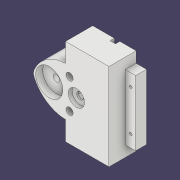
# Autodesk Inventor part: AA006b
Saved by Autodesk Inventor 2017 SP1 (Build 210196100, 196)
## iProperties
Created: 2017-06-04
Part Number: AA006b
Material: ABS Plastic
Document SubType Name: Modeling
Designer: Zach
Density: 1.06 g/cm^3
Appearance: CR White
Author: Zach
Autodesk Inventor part; units mm, degrees
ref_plane "YZ Plane" through (0, 0, 0) normal (1, 0, 0) x (0, 1, 0)
ref_plane "XZ Plane" through (0, 0, 0) normal (0, 1, 0) x (-1, 0, 0)
ref_plane "XY Plane" through (0, 0, 0) normal (0, 0, 1) x (1, 0, 0)
sketch "Sketch1" plane through (0, 0, 0) normal (0, 0, 1) x (1, 0, 0)
  line L0 (0, 0) -> (160, 0)
  line L1 (160, 0) -> (160, 160)
  line L2 (160, 160) -> (0, 160)
  line L3 (0, 160) -> (0, 0)
  circle A0 centre (50, 80) radius 6
  point P0 (160, 80)
  dimension "d0" = 160
  dimension "d1" = 160
  dimension "d2" = 12
  dimension "d7" = 50
  constraints: 8 end point, 2 parallel, 1 centre point, 1 horizontal, 1 horizontal alignment, 1 midpoint, 1 perpendicular
  measures "d0" distance of L2.end L1.end
  measures "d1" distance of L1.end L0.end
  measures "d2" diameter of A0
  measures "d7" distance from line of L3 A0.centre
extrude "Extrusion1" add sketch "Sketch1" along normal blind 50
sketch "Sketch5" plane through (0, 0, 50) normal (0, 0, 1) x (1, 0, 0)
  circle A0 centre (50, 80) radius 6 projected
  line L0 (0, 0) -> (160, 0) projected
  line L1 (160, 0) -> (160, 160) projected
  line L2 (160, 160) -> (0, 160) projected
  line L3 (0, 160) -> (0, 0) projected
  circle A1 centre (80, 80) radius 80 construction
  line L4 (0, 0) -> (160, 0) projected
  arc A2 (80, 160) -> (80, 0) centre (80, 80) ccw
  line L5 (160, 160) -> (0, 160) projected
  line L6 (80, 160) -> (0, 160)
  line L7 (0, 160) -> (0, 0)
  line L8 (80, 0) -> (0, 0)
  point P0 (0, 80)
  constraints: 6 end point, 4 point on circle, 4 tangent, 3 midpoint, 2 centre point, 2 collinear, 1 horizontal alignment, 1 perpendicular
extrude "Extrusion5" cut sketch "Sketch5" against normal through all contours L3 A2 L0 | L3 L2 A2
sketch "Sketch17" plane through (0, 0, 50) normal (0, 0, 1) x (1, 0, 0)
  circle A0 centre (50, 80) radius 6 projected
  circle A1 centre (50, 80) radius 6 projected
  circle A2 centre (50, 80) radius 25
  point P0 (0, 0)
  dimension "d80" = 50
  constraints: 1 centre point, 1 coincident
  measures "d80" diameter of A2
extrude "Extrusion17" cut sketch "Sketch17" against normal blind 10
sketch "Sketch18" plane through (0, 0, 0) normal (0, 0, -1) x (-1, 0, 0)
  circle A0 centre (-50, 80) radius 6 projected
  point P0 (0, 0)
extrude "Extrusion18" add sketch "Sketch18" against normal blind 12.5
sketch "Sketch19" plane through (0, 0, 0) normal (0, 0, -1) x (-1, 0, 0)
  line L0 (-160, 0) -> (-160, 160) projected
  line L1 (-160, 20) -> (-179, 20)
  line L2 (-179, 20) -> (-179, 140)
  line L3 (-179, 140) -> (-160, 140)
  line L4 (-160, 140) -> (-160, 20)
  line L5 (-80, 0) -> (-160, 0) projected
  line L6 (-160, 160) -> (-80, 160) projected
  circle A0 centre (-170, 42.5) radius 2.5
  line L7 (-170, 42.5) -> (-170, 117.5) construction
  circle A1 centre (-170, 117.5) radius 2.5
  point P0 (0, 0)
  point P1 (-160, 80)
  point P2 (-170, 80)
  point P3 (-160, 80)
  dimension "d85" = 19
  dimension "d86" = 20
  dimension "d87" = 20
  dimension "d88" = 5
  dimension "d89" = 10
  dimension "d100" = 75
  dimension "d101" = 5
  constraints: 10 end point, 3 midpoint, 2 centre point, 2 parallel, 1 coincident, 1 horizontal, 1 horizontal alignment, 1 perpendicular, 1 point on line, 1 vertical
  measures "d85" distance of L2.end L3.end
  measures "d86" distance between parallel lines of L1 L5
  measures "d87" distance between parallel lines of L6 L3
  measures "d88" diameter of A0
  measures "d89" distance from line of L0 L7.start
  measures "d100" distance of L7.start L7.end
  measures "d101" diameter of A1
extrude "Extrusion19" add sketch "Sketch19" against normal blind 20
sketch "Sketch20" plane through (0, 0, 0) normal (0, 0, -1) x (-1, 0, 0)
  circle A0 centre (-170, 42.5) radius 2.5 projected
  circle A1 centre (-170, 42.5) radius 6.5
  circle A2 centre (-170, 117.5) radius 2.5 projected
  circle A3 centre (-170, 117.5) radius 6.5
  point P0 (0, 0)
  dimension "d92" = 13
  dimension "d102" = 13
  constraints: 2 centre point, 2 coincident
  measures "d92" diameter of A1
  measures "d102" diameter of A3
extrude "Extrusion20" cut sketch "Sketch20" against normal blind 15 contours A0 | A1 | A3
sketch "Sketch21" plane through (0, 0, 0) normal (0, 0, -1) x (-1, 0, 0)
  circle A0 centre (-170, 42.5) radius 6.5 projected
  arc A1 (-80, 0) -> (-80, 160) centre (-80, 80) ccw projected
  line L0 (-160, 160) -> (-80, 160) projected
  line L1 (-160, 140) -> (-160, 160) projected
  line L2 (-179, 140) -> (-160, 140) projected
  line L3 (-179, 20) -> (-179, 140) projected
  line L4 (-160, 20) -> (-179, 20) projected
  line L5 (-160, 0) -> (-160, 20) projected
  line L6 (-80, 0) -> (-160, 0) projected
  circle A2 centre (-50, 80) radius 6 construction
  arc A3 (-80, 10) -> (-80, 150) centre (-80, 80) ccw construction
  line L7 (-80, 10) -> (-150, 10)
  line L8 (-150, 10) -> (-150, 30)
  line L9 (-150, 30) -> (-169, 30) construction
  line L10 (-169, 30) -> (-169, 130) construction
  line L11 (-169, 130) -> (-150, 130) construction
  line L12 (-150, 130) -> (-150, 150)
  line L13 (-150, 150) -> (-80, 150)
  line L14 (-150, 130) -> (-150, 30) construction
  line L15 (-150, 72.5) -> (-73.8485, 72.5)
  line L16 (-111.9242, 72.5) -> (-111.9242, 87.5) construction
  line L17 (-150, 87.5) -> (-73.8485, 87.5)
  line L18 (-150, 130) -> (-150, 87.5)
  line L19 (-150, 30) -> (-150, 72.5)
  line L20 (-26.1515, 72.5) -> (-10.4029, 72.5)
  line L21 (-26.1515, 87.5) -> (-10.4029, 87.5)
  line L22 (-57.5, 103.8485) -> (-57.5, 146.2854)
  line L23 (-42.5, 103.8485) -> (-42.5, 139.108)
  line L24 (-57.5, 121.4782) -> (-42.5, 121.4782) construction
  line L25 (-42.5, 56.1515) -> (-42.5, 20.892)
  line L26 (-57.5, 56.1515) -> (-57.5, 13.7146)
  circle A4 centre (-50, 80) radius 25 construction
  arc A5 (-57.5, 146.2854) -> (-80, 150) centre (-80, 80) ccw
  arc A6 (-10.4029, 87.5) -> (-42.5, 139.108) centre (-80, 80) ccw
  arc A7 (-42.5, 20.892) -> (-10.4029, 72.5) centre (-80, 80) ccw
  arc A8 (-80, 10) -> (-57.5, 13.7146) centre (-80, 80) ccw
  arc A9 (-57.5, 103.8485) -> (-73.8485, 87.5) centre (-50, 80) ccw
  arc A10 (-26.1515, 87.5) -> (-42.5, 103.8485) centre (-50, 80) ccw
  arc A11 (-42.5, 56.1515) -> (-26.1515, 72.5) centre (-50, 80) ccw
  arc A12 (-73.8485, 72.5) -> (-57.5, 56.1515) centre (-50, 80) ccw
  point P0 (0, 0)
  point P1 (-111.9242, 80)
  point P2 (-50, 121.4782)
  dimension "d95" = 10
  dimension "d96" = 15
  dimension "d99" = 15
  constraints: 40 end point, 27 point on circle, 9 centre point, 9 concentric, 5 midpoint, 5 vertical, 3 horizontal, 3 horizontal alignment, 3 point on line, 3 vertical alignment, 2 collinear, 2 parallel, 1 perpendicular, 7 other
  measures "d95" distance between parallel lines of L0 L13
  measures "d96" distance of L16.end L16.start
  measures "d99" distance of L24.end L24.start
extrude "Extrusion21" cut sketch "Sketch21" against normal blind 40 contours L7 L8 L19 L15 A12 L26 A8 | L12 L13 A5 L22 A9 L17 L18 | L20 A7 L25 A11 | A10 L23 A6 L21
sketch "Sketch23" plane through (0, 0, 50) normal (0, 0, 1) x (1, 0, 0)
  circle A0 centre (87.5, 52.5) radius 2.5
  circle A1 centre (87.5, 107.5) radius 2.5
  line L0 (160, 0) -> (160, 160) construction
  line L1 (87.5, 52.5) -> (87.5, 107.5) construction
  point P0 (0, 0)
  point P1 (87.5, 80)
  point P2 (160, 80)
  dimension "d103" = 5
  dimension "d104" = 5
  dimension "d105" = 55
  dimension "d106" = 72.5
  constraints: 2 centre point, 2 end point, 2 midpoint, 1 horizontal alignment, 1 vertical, 1 vertical alignment
  measures "d103" diameter of A0
  measures "d104" diameter of A1
  measures "d105" distance of L1.start L1.end
  measures "d106" distance from line of L0 L1.start
extrude "Extrusion22" cut sketch "Sketch23" against normal through all
sketch "Sketch24" plane through (0, 0, 40) normal (0, 0, -1) x (-1, 0, 0)
  line L0 (-95, 150) -> (-95, 10)
  line L1 (-80, 150) -> (-80, 10)
  line L2 (-80, 150) -> (-95, 150)
  line L3 (-95, 10) -> (-80, 10)
  line L4 (-95, 80) -> (-80, 80) construction
  circle A0 centre (-87.5, 107.5) radius 2.5 projected
  circle A1 centre (-87.5, 52.5) radius 2.5 projected
  point P0 (0, 0)
  point P1 (-87.5, 80)
  point P2 (-87.5, 10)
  point P3 (-150, 150)
  point P4 (-150, 10)
  dimension "d110" = 15
  constraints: 10 end point, 4 horizontal alignment, 4 midpoint, 2 horizontal, 2 vertical, 1 vertical alignment
  measures "d110" distance of L4.start L4.end
extrude "Extrusion23" add sketch "Sketch24" along normal blind 40
sketch "Sketch26" plane through (0, 0, 50) normal (0, 0, 1) x (1, 0, 0)
  circle A0 centre (87.5, 107.5) radius 2.5 projected
  circle A1 centre (87.5, 52.5) radius 2.5 projected
  circle A2 centre (87.5, 52.5) radius 6.5
  circle A3 centre (87.5, 107.5) radius 6.5
  point P0 (0, 0)
  dimension "d115" = 13
  dimension "d116" = 13
  constraints: 2 centre point, 2 coincident
  measures "d115" diameter of A2
  measures "d116" diameter of A3
extrude "Extrusion24" cut sketch "Sketch26" against normal blind 30 contours A0 | A1 | A2 | A3
sketch "Sketch27" plane through (0, 0, 50) normal (0, 0, 1) x (1, 0, 0)
  arc A0 (80, 160) -> (80, 0) centre (80, 80) ccw construction
  circle A1 centre (80, 80) radius 80 construction
  circle A2 centre (80, 80) radius 60 construction
  line L0 (80, 0) -> (160, 0) projected
  line L1 (160, 160) -> (80, 160) projected
  arc A3 (80, 160) -> (80, 0) centre (80, 80) ccw projected
  arc A4 (80, 160) -> (80, 160) centre (80, 80) ccw
  line L2 (80, 160) -> (80, 140)
  line L3 (160, 0) -> (122.4264, 37.5736)
  line L4 (160, 0) -> (80, 80) construction
  arc A5 (80, 140) -> (122.4264, 37.5736) centre (80, 80) ccw
  circle A6 centre (50, 80) radius 6 projected
  arc A7 (80, 160) -> (80, 0) centre (80, 80) ccw projected
  point P0 (0, 0)
  dimension "d119" = 20
  constraints: 6 end point, 6 point on circle, 3 centre point, 2 coincident, 2 concentric, 2 vertical alignment, 1 point on line, 1 vertical, 6 other
extrude "Extrusion25" cut sketch "Sketch27" against normal blind 25 contours A4 L3 L0 | A3 L2 A5 L3 A4
sketch "Sketch30" plane through (0, 0, 25) normal (0, 0, 1) x (1, 0, 0)
  line L0 (95, 21.9052) -> (95, 10)
  line L1 (122.4264, 37.5736) -> (160, 0) construction
  arc A0 (95, 21.9052) -> (122.4264, 37.5736) centre (80, 80) ccw
  line L2 (150, 10) -> (122.4264, 37.5736)
  arc A1 (80, 140) -> (122.4264, 37.5736) centre (80, 80) ccw projected
  line L3 (95, 10) -> (150, 10) projected
  line L4 (95, 10) -> (150, 10) projected
  point P0 (0, 0)
  constraints: 6 end point, 2 point on circle, 1 centre point, 1 concentric, 1 point on line, 1 vertical
extrude "Extrusion28" add sketch "Sketch30" against normal blind 5
sketch "Sketch31" plane through (0, 0, 25) normal (0, 0, 1) x (1, 0, 0)
  arc A0 (10.4029, 72.5) -> (42.5, 20.892) centre (80, 80) ccw projected
  line L0 (80, 87.5) -> (80, 150) projected
  arc A1 (57.5, 13.7146) -> (80, 10) centre (80, 80) ccw projected
  line L1 (26.1515, 72.5) -> (10.4029, 72.5) projected
  arc A2 (80, 150) -> (80, 10) centre (80, 80) ccw
  arc A3 (80, 140) -> (122.4264, 37.5736) centre (80, 80) ccw projected
  line L2 (80, 10) -> (80, 20)
  line L3 (80, 150) -> (80, 140)
  line L4 (80, 140) -> (80, 20)
  arc A4 (80, 140) -> (80, 20) centre (80, 80) ccw
  constraints: 6 end point, 6 point on circle, 2 centre point, 2 vertical, 1 collinear, 1 concentric
extrude "Extrusion29" add sketch "Sketch31" against normal blind 10 contours L1 A3 L2 A1 A2 A0 | A2 L0 A3 L1
sketch "Sketch32" plane through (0, 0, 40) normal (0, 0, -1) x (-1, 0, 0)
  arc A0 (-122.4264, 37.5736) -> (-80, 140) centre (-80, 80) ccw construction
  line L0 (-122.4264, 37.5736) -> (-160, 0) construction
  line L1 (-160, 0) -> (-160, 160) construction
  arc A1 (-122.2654, 44.8057) -> (-80, 135) centre (-80, 80) ccw construction
  line L2 (-122.2654, 44.8057) -> (-155, 12.0711) construction
  line L3 (-155, 12.0711) -> (-155, 160) construction
  line L4 (-150, 10) -> (-150, 72.5) construction
  arc A2 (-122.4264, 37.5736) -> (-80, 140) centre (-80, 80) ccw
  arc A3 (-122.2654, 44.8057) -> (-80, 135) centre (-80, 80) ccw
  line L5 (-122.2654, 44.8057) -> (-150, 17.0711)
  line L6 (-150, 10) -> (-150, 17.0711)
  line L7 (-150, 10) -> (-122.4264, 37.5736)
  line L8 (-80, 140) -> (-80, 135)
  point P0 (0, 0)
  dimension "d155" = 5
  constraints: 12 end point, 6 point on circle, 3 centre point, 2 collinear, 2 concentric, 2 point on line, 1 parallel, 2 other
  measures "d155" radial gap between concentric circles of A0 A1
extrude "Extrusion30" add sketch "Sketch32" along normal blind 25
sketch "Sketch33" plane through (0, 0, 20) normal (0, 0, -1) x (-1, 0, 0)
  line L0 (-95, 10) -> (-150, 10) projected
  line L1 (-95, 21.9052) -> (-95, 10) projected
  arc A0 (-122.4264, 37.5736) -> (-95, 21.9052) centre (-80, 80) ccw projected
  line L2 (-122.4264, 37.5736) -> (-150, 10) projected
  point P0 (0, 0)
extrude "Extrusion31" add sketch "Sketch33" along normal blind 5
sketch "Sketch34" plane through (0, 0, 50) normal (0, 0, 1) x (1, 0, 0)
  circle A0 centre (100, 80) radius 6.5
  circle A1 centre (50, 80) radius 6 projected
  point P0 (0, 0)
  dimension "d143" = 13
  dimension "d144" = 50
  constraints: 1 centre point, 1 horizontal alignment
  measures "d143" diameter of A0
  measures "d144" distance of A0.centre A1.centre
extrude "Extrusion32" cut sketch "Sketch34" against normal through all contours A0
sketch "Sketch35" plane through (0, 0, 40) normal (0, 0, -1) x (-1, 0, 0)
  line L0 (-88, 94.5) -> (-112, 94.5)
  line L1 (-112, 94.5) -> (-112, 65.5)
  line L2 (-112, 65.5) -> (-88, 65.5)
  line L3 (-88, 65.5) -> (-88, 94.5)
  circle A0 centre (-100, 80) radius 6.5 projected
  line L4 (-95, 55.5) -> (-150, 55.5)
  line L5 (-150, 55.5) -> (-150, 104.5)
  line L6 (-150, 104.5) -> (-95, 104.5)
  line L7 (-95, 104.5) -> (-95, 55.5)
  line L8 (-150, 10) -> (-150, 72.5) projected
  line L9 (-95, 72.5) -> (-95, 10) projected
  point P0 (0, 0)
  point P1 (-88, 80)
  point P2 (-100, 65.5)
  dimension "d147" = 29
  dimension "d148" = 24
  dimension "d153" = 10
  dimension "d154" = 10
  constraints: 16 end point, 4 parallel, 2 midpoint, 2 perpendicular, 2 point on line, 1 horizontal, 1 horizontal alignment, 1 vertical alignment
  measures "d147" distance of L2.end L0.start
  measures "d148" distance of L1.end L2.end
  measures "d153" distance between parallel lines of L4 L2
  measures "d154" distance between parallel lines of L0 L6
extrude "Extrusion33" add sketch "Sketch35" along normal blind 40 contours L0 L1 L2 L7 L4 L5 L6
sketch "Sketch36" plane through (0, 0, 40) normal (0, 0, -1) x (-1, 0, 0)
  line L0 (-112, 94.5) -> (-112, 87.5) construction
  line L1 (-73.8485, 87.5) -> (-80, 87.5) construction
  line L2 (-95, 94.5) -> (-112, 94.5) construction
  line L3 (-112, 72.5) -> (-112, 65.5) construction
  line L4 (-112, 65.5) -> (-95, 65.5) construction
  line L5 (-80, 72.5) -> (-73.8485, 72.5) construction
  line L6 (-88, 94.5) -> (-112, 94.5)
  line L7 (-112, 94.5) -> (-112, 65.5)
  line L8 (-112, 65.5) -> (-88, 65.5)
  line L9 (-88, 65.5) -> (-88, 94.5)
  line L10 (-57.5, 56.1515) -> (-57.5, 29.8129) projected
  arc A0 (-73.8485, 72.5) -> (-57.5, 56.1515) centre (-50, 80) ccw projected
  line L11 (-80, 72.5) -> (-80, 25) projected
  line L12 (-95, 65.5) -> (-95, 72.5) projected
  line L13 (-112, 72.5) -> (-95, 72.5) projected
  line L14 (-80, 135) -> (-80, 87.5) projected
  arc A1 (-57.5, 103.8485) -> (-73.8485, 87.5) centre (-50, 80) ccw projected
  line L15 (-57.5, 130.1871) -> (-57.5, 103.8485) projected
  line L16 (-95, 87.5) -> (-112, 87.5) projected
  line L17 (-95, 87.5) -> (-95, 94.5) projected
  line L18 (-57.5, 56.1515) -> (-57.5, 29.8129) projected
  arc A2 (-73.8485, 72.5) -> (-57.5, 56.1515) centre (-50, 80) ccw projected
  line L19 (-80, 72.5) -> (-73.8485, 72.5) projected
  arc A3 (-80, 25) -> (-57.5, 29.8129) centre (-80, 80) ccw projected
  arc A4 (-57.5, 130.1871) -> (-80, 135) centre (-80, 80) ccw projected
  arc A5 (-80, 25) -> (-57.5, 29.8129) centre (-80, 80) ccw projected
  line L20 (-80, 72.5) -> (-80, 25) projected
  point P0 (0, 0)
  constraints: 8 end point, 2 parallel, 1 horizontal, 1 perpendicular
extrude "Extrusion34" cut sketch "Sketch36" along normal through all contours L9 L8 L12 L13 L7 L16 L17 L6 | L17 L16 L7 L6 | L8 L7 L13 L12
sketch "Sketch37" plane through (0, 0, 50) normal (0, 0, 1) x (1, 0, 0)
  circle A0 centre (50, 80) radius 6 projected
  arc A1 (80, 140) -> (122.4264, 37.5736) centre (80, 80) ccw construction
  arc A2 (80, 125) -> (20, 80) centre (81.8551, 60.0265) ccw
  line L0 (80, 140) -> (80, 125)
  line L1 (80, 135) -> (80, 87.5) projected
  arc A3 (80, 140) -> (20, 80) centre (80, 80) ccw
  arc A4 (20, 80) -> (115.3553, 44.6447) centre (81.7535, 100.2856) ccw
  arc A5 (20, 80) -> (122.4264, 37.5736) centre (80, 80) ccw
  line L2 (122.4264, 37.5736) -> (115.3553, 44.6447)
  line L3 (122.4264, 37.5736) -> (160, 0) construction
  point P0 (0, 0)
  dimension "d156" = 15
  dimension "d157" = 65
  dimension "d158" = 65
  dimension "d159" = 10
  constraints: 9 point on circle, 4 centre point, 4 end point, 3 concentric, 2 collinear, 1 horizontal alignment, 1 vertical alignment
  measures "d156" distance of L0.start L0.end
  measures "d157" radius of A2
  measures "d158" radius of A4
  measures "d159" distance of L2.start L2.end
extrude "Extrusion35" cut sketch "Sketch37" against normal blind 25 contours A4 L2 A5 | A2 A3 L0
sketch "Sketch38" plane through (0, 0, 50) normal (0, 0, 1) x (1, 0, 0)
  line L0 (80, 160) -> (80, 125) projected
  arc A0 (20, 80) -> (115.3553, 44.6447) centre (81.7535, 100.2856) ccw construction
  arc A1 (80, 35.3093) -> (115.3553, 44.6447) centre (81.7535, 100.2856) ccw
  line L1 (115.3553, 44.6447) -> (160, 0)
  line L2 (160, 0) -> (80, 0) projected
  line L3 (80, 72.5) -> (80, 35.3093) projected
  line L4 (80, 35.3093) -> (80, 0)
  point P0 (0, 0)
  constraints: 4 end point, 3 point on circle, 1 centre point, 1 collinear, 1 concentric, 1 vertical alignment
extrude "Extrusion36" add sketch "Sketch38" against normal blind 25
sketch "Sketch39" plane through (0, 0, 40) normal (0, 0, -1) x (-1, 0, 0)
  arc A0 (-80, 35.3093) -> (-20, 80) centre (-81.7535, 100.2856) ccw projected
  arc A1 (-20, 80) -> (-80, 125) centre (-81.8551, 60.0265) ccw projected
  arc A2 (-25.282, 80.0133) -> (-80, 119.9978) centre (-81.8551, 60.0265) ccw
  arc A3 (-80, 40.3112) -> (-25.282, 80.0133) centre (-81.7535, 100.2856) ccw
  line L0 (-80, 125) -> (-80, 119.9978)
  line L1 (-80, 35.3093) -> (-80, -5) projected
  line L2 (-80, 40.3112) -> (-80, 35.3093)
  point P0 (0, 0)
  dimension "d164" = 5
  constraints: 4 end point, 4 point on circle, 2 centre point, 2 vertical, 1 other
  measures "d164" radial gap between concentric circles of A1 A2
extrude "Extrusion37" add sketch "Sketch39" along normal blind 25
sketch "Sketch42" plane through (0, 0, 25) normal (0, 0, 1) x (1, 0, 0)
  arc A0 (80, 125) -> (20, 80) centre (81.8551, 60.0265) ccw projected
  arc A1 (20, 80) -> (80, 35.3093) centre (81.7535, 100.2856) ccw projected
  arc A2 (80, 135) -> (57.5, 130.1871) centre (80, 80) ccw projected
  line L0 (80, 0) -> (80, 25) projected
  arc A3 (57.5, 29.8129) -> (80, 25) centre (80, 80) ccw projected
  line L1 (57.5, 39.98) -> (57.5, 29.8129) projected
  arc A4 (42.5, 48.4767) -> (57.5, 39.98) centre (81.7535, 100.2856) ccw projected
  line L2 (42.5, 39.7663) -> (42.5, 48.4767) projected
  arc A5 (27.023, 65.2203) -> (42.5, 39.7663) centre (80, 80) ccw projected
  arc A6 (20, 80) -> (27.023, 65.2203) centre (81.7535, 100.2856) ccw projected
  arc A7 (27.1002, 95.0535) -> (20, 80) centre (81.8551, 60.0265) ccw projected
  arc A8 (42.5, 120.2337) -> (27.1002, 95.0535) centre (80, 80) ccw projected
  line L3 (42.5, 111.7582) -> (42.5, 120.2337) projected
  arc A9 (57.5, 120.2911) -> (42.5, 111.7582) centre (81.8551, 60.0265) ccw projected
  line L4 (57.5, 130.1871) -> (57.5, 120.2911) projected
  arc A10 (80, 135) -> (57.5, 130.1871) centre (80, 80) ccw projected
  line L5 (80, 160) -> (80, 135) projected
  arc A11 (80, 160) -> (80, 0) centre (80, 80) ccw projected
  line L6 (80, 135) -> (80, 125)
  arc A12 (57.5, 39.98) -> (80, 35.3093) centre (81.7535, 100.2856) ccw projected
  line L7 (80, 25) -> (80, 35.3093)
  line L8 (80, 10) -> (80, 72.5) projected
  point P0 (0, 0)
  constraints: 4 end point, 1 collinear, 1 vertical
extrude "Extrusion38" add sketch "Sketch42" against normal blind 5
sketch "Sketch43" plane through (0, 0, 15) normal (0, 0, -1) x (-1, 0, 0)
  arc A0 (-119.618, 47.4531) -> (-80, 35.3093) centre (-81.7535, 100.2856) ccw
  arc A1 (-122.2654, 44.8057) -> (-118.8909, 41.1091) centre (-80, 80) ccw projected
  line L0 (-122.2654, 44.8057) -> (-119.618, 47.4531)
  line L1 (-122.2654, 44.8057) -> (-150, 17.0711) projected
  arc A2 (-42.5, 39.7663) -> (-27.023, 65.2203) centre (-80, 80) ccw projected
  arc A3 (-122.2654, 44.8057) -> (-27.023, 65.2203) centre (-80, 80) ccw
  arc A4 (-27.1002, 95.0535) -> (-42.5, 120.2337) centre (-80, 80) ccw projected
  line L2 (-42.5, 111.7582) -> (-42.5, 120.2337) projected
  arc A5 (-27.1002, 95.0535) -> (-42.5, 111.7582) centre (-81.8551, 60.0265) ccw projected
  arc A6 (-57.5, 130.1871) -> (-80, 135) centre (-80, 80) ccw projected
  line L3 (-80, 125) -> (-80, 135) projected
  arc A7 (-57.5, 120.2911) -> (-80, 125) centre (-81.8551, 60.0265) ccw projected
  line L4 (-57.5, 130.1871) -> (-57.5, 120.2911) projected
  arc A8 (-80, 35.3093) -> (-20, 80) centre (-81.7535, 100.2856) ccw projected
  arc A9 (-115.3553, 44.6447) -> (-95, 36.6497) centre (-81.7535, 100.2856) ccw projected
  arc A10 (-80, 35.3093) -> (-27.023, 65.2203) centre (-81.7535, 100.2856) ccw
  point P0 (0, 0)
  constraints: 7 point on circle, 3 centre point, 3 concentric, 2 end point, 1 collinear
extrude "Extrusion39" add sketch "Sketch43" against normal blind 10
sketch "Sketch44" plane through (0, 0, 40) normal (0, 0, -1) x (-1, 0, 0)
  line L0 (-118.8909, 41.1091) -> (-115.3553, 44.6447) projected
  arc A0 (-115.3553, 44.6447) -> (-95, 36.6497) centre (-81.7535, 100.2856) ccw construction
  line L1 (-95, 36.6497) -> (-95, 55.5) construction
  line L2 (-95, 55.5) -> (-150, 55.5) construction
  line L3 (-150, 17.0711) -> (-150, 55.5) construction
  line L4 (-150, 17.0711) -> (-122.2654, 44.8057) construction
  arc A1 (-122.2654, 44.8057) -> (-118.8909, 41.1091) centre (-80, 80) ccw projected
  arc A2 (-119.618, 47.4531) -> (-95, 36.6497) centre (-81.7535, 100.2856) ccw construction
  line L5 (-119.618, 47.4531) -> (-150, 17.0711) construction
  arc A3 (-119.618, 47.4531) -> (-115.3553, 44.6447) centre (-81.7535, 100.2856) ccw
  line L6 (-119.618, 47.4531) -> (-122.2654, 44.8057)
  point P0 (0, 0)
  constraints: 2 end point, 2 point on circle, 1 centre point, 1 concentric
extrude "Extrusion40" add sketch "Sketch44" along normal blind 15
fillet "Fillet1" radius 15 2 edges at (20, 80, 45) (20, 80, 32.5)
sketch "Sketch45" plane through (0, 0, 40) normal (0, 0, -1) x (-1, 0, 0)
  line L0 (-95, 55.5) -> (-95, 10) projected
  line L1 (-95, 10) -> (-150, 10) projected
  line L2 (-150, 10) -> (-150, 55.5) projected
  line L3 (-150, 55.5) -> (-95, 55.5) projected
  point P0 (0, 0)
extrude "Extrusion41" cut sketch "Sketch45" along normal through all
sketch "Sketch47" plane through (80, 160, 25) normal (-1, 0, 0) x (0, 0, 1)
  line L0 (7, -10) -> (0, -10)
  line L1 (0, -10) -> (0, -25)
  line L2 (0, -25) -> (7, -25)
  line L3 (7, -25) -> (7, -10)
  line L4 (0, 0) -> (0, -160) projected
  line L5 (0, 0) -> (0, -35) projected
  line L6 (7, -134.8454) -> (0, -134.8454)
  line L7 (0, -134.8454) -> (0, -149.8454)
  line L8 (0, -149.8454) -> (7, -149.8454)
  line L9 (7, -149.8454) -> (7, -134.8454)
  line L10 (0, -124.6907) -> (0, -160) projected
  point P0 (-25, -160)
  point P1 (0, -17.5)
  point P2 (0, -142.3454)
  dimension "d185" = 7
  dimension "d186" = 15
  dimension "d188" = 7
  dimension "d189" = 15
  constraints: 16 end point, 4 midpoint, 4 parallel, 2 horizontal, 2 perpendicular
  measures "d185" distance of L2.end L1.end
  measures "d186" distance of L1.end L0.end
  measures "d188" distance of L8.end L7.end
  measures "d189" distance of L7.end L6.end
extrude "Extrusion43" cut sketch "Sketch47" against normal blind 15
sketch "Sketch48" plane through (160, 160, 50) normal (0, 1, 0) x (1, 0, 0)
  line L0 (-40, 42) -> (-30, 42)
  line L1 (-30, 42) -> (-30, 50)
  line L2 (-30, 50) -> (-40, 50)
  line L3 (-40, 50) -> (-40, 42)
  line L4 (0, 50) -> (0, 0) projected
  line L5 (0, 50) -> (-80, 50) projected
  point P0 (-160, 50)
  dimension "d192" = 10
  dimension "d193" = 8
  dimension "d202" = 30
  constraints: 8 end point, 2 parallel, 1 horizontal, 1 midpoint, 1 perpendicular
  measures "d192" distance of L2.end L1.end
  measures "d193" distance of L1.end L0.end
  measures "d202" distance between parallel lines of L4 L1
extrude "Extrusion44" cut sketch "Sketch48" against normal blind 15
sketch "Sketch49" plane through (160, 0, 0) normal (0, -1, 0) x (1, 0, 0)
  line L0 (-30, 0) -> (-30, 8) construction
  line L1 (-30, 8) -> (-40, 8) construction
  line L2 (-40, 8) -> (-40, 0) construction
  line L3 (-80, 0) -> (-80, 25) construction
  line L4 (-80, 25) -> (-80, 50) construction
  line L5 (0, 50) -> (-80, 50) construction
  line L6 (0, 0) -> (0, 50) construction
  line L7 (0, 0) -> (-30, 0) construction
  line L8 (-40, 0) -> (-80, 0) construction
  line L9 (-40, 8) -> (-30, 8)
  line L10 (-30, 8) -> (-30, 0)
  line L11 (-30, 0) -> (-40, 0)
  line L12 (-40, 0) -> (-40, 8)
  point P0 (-160, 0)
  constraints: 8 end point, 2 parallel, 1 horizontal, 1 perpendicular
extrude "Extrusion45" cut sketch "Sketch49" against normal blind 15
sketch "Sketch50" plane through (0, 0, 40) normal (0, 0, 1) x (1, 0, 0)
  arc A0 (39.8068, 102.8276) -> (40.2057, 56.9985) centre (50, 80) ccw projected
  arc A1 (40.2057, 56.9985) -> (42.5, 56.1515) centre (50, 80) ccw projected
  arc A2 (42.5, 56.1515) -> (57.5, 56.1515) centre (50, 80) ccw projected
  arc A3 (57.5, 56.1515) -> (73.8485, 72.5) centre (50, 80) ccw projected
  arc A4 (73.8485, 72.5) -> (73.8485, 87.5) centre (50, 80) ccw projected
  arc A5 (73.8485, 87.5) -> (57.5, 103.8485) centre (50, 80) ccw projected
  arc A6 (57.5, 103.8485) -> (42.5, 103.8485) centre (50, 80) ccw projected
  arc A7 (42.5, 103.8485) -> (39.8068, 102.8276) centre (50, 80) ccw projected
  circle A8 centre (50, 80) radius 6 projected
  point P0 (0, 0)
extrude "Extrusion46" cut sketch "Sketch50" against normal blind 3
sketch "Sketch51" plane through (0, 0, 40) normal (0, 0, -1) x (-1, 0, 0)
  arc A0 (-39.8068, 102.8276) -> (-42.5, 105.3164) centre (-81.8551, 60.0265) ccw projected
  line L0 (-42.5, 103.8485) -> (-42.5, 105.3164) projected
  arc A1 (-39.8068, 102.8276) -> (-42.5, 103.8485) centre (-50, 80) ccw projected
  arc A2 (-42.5, 54.9076) -> (-40.2057, 56.9985) centre (-81.7535, 100.2856) ccw projected
  arc A3 (-42.5, 56.1515) -> (-40.2057, 56.9985) centre (-50, 80) ccw projected
  line L1 (-42.5, 54.9076) -> (-42.5, 56.1515) projected
  arc A4 (-80, 40.3112) -> (-57.5, 45.406) centre (-81.7535, 100.2856) ccw projected
  line L2 (-57.5, 56.1515) -> (-57.5, 45.406) projected
  arc A5 (-73.8485, 72.5) -> (-57.5, 56.1515) centre (-50, 80) ccw projected
  line L3 (-80, 72.5) -> (-73.8485, 72.5) projected
  line L4 (-80, 72.5) -> (-80, 40.3112) projected
  arc A6 (-57.5, 114.861) -> (-80, 119.9978) centre (-81.8551, 60.0265) ccw projected
  line L5 (-80, 119.9978) -> (-80, 87.5) projected
  line L6 (-73.8485, 87.5) -> (-80, 87.5) projected
  arc A7 (-57.5, 103.8485) -> (-73.8485, 87.5) centre (-50, 80) ccw projected
  line L7 (-57.5, 114.861) -> (-57.5, 103.8485) projected
  point P0 (0, 0)
extrude "Extrusion47" add sketch "Sketch51" along normal blind 25
sketch "Sketch52" plane through (95, 104.5, 40) normal (0, 1, 0) x (1, 0, 0)
  line L0 (55, 0) -> (0, 0) construction
  line L1 (55, 40) -> (55, 0) construction
  line L2 (0, 40) -> (55, 40) construction
  line L3 (0, 0) -> (0, 40) construction
  line L4 (17, 0) -> (-7, 0) construction
  line L5 (17, 0) -> (17, 40) construction
  line L6 (-7, 40) -> (17, 40) construction
  line L7 (-7, 0) -> (-7, 40) construction
  line L8 (1, 40) -> (16, 40)
  line L9 (16, 40) -> (16, 30)
  line L10 (16, 30) -> (1, 30)
  line L11 (1, 30) -> (1, 40)
  line L12 (0, 40) -> (17, 40)
  point P0 (-95, 40)
  point P1 (8.5, 40)
  point P2 (8.5, 40)
  dimension "d204" = 15
  dimension "d205" = 10
  constraints: 10 end point, 2 midpoint, 2 parallel, 1 coincident, 1 collinear, 1 horizontal, 1 perpendicular, 1 point on line
  measures "d204" distance of L9.end L10.end
  measures "d205" distance of L8.end L9.end
extrude "Extrusion48" cut sketch "Sketch52" against normal blind 49
sketch "Sketch53" plane through (0, 0, 25) normal (0, 0, 1) x (1, 0, 0)
  arc A0 (80, 125) -> (22.2896, 86.0447) centre (81.8551, 60.0265) ccw projected
  line L0 (80, 135) -> (80, 125) projected
  line L1 (80, 135) -> (95, 135) projected
  line L2 (95, 150) -> (95, 135) projected
  line L3 (80, 150) -> (95, 150) projected
  line L4 (80, 160) -> (80, 150) projected
  arc A1 (80, 160) -> (80, 0) centre (80, 80) ccw projected
  line L5 (80, 10.1546) -> (80, 0) projected
  line L6 (80, 10.1546) -> (95, 10.1546) projected
  line L7 (95, 25.1546) -> (95, 10.1546) projected
  line L8 (80, 25.1546) -> (95, 25.1546) projected
  line L9 (80, 35.3093) -> (80, 25.1546) projected
  arc A2 (22.3201, 73.9669) -> (80, 35.3093) centre (81.7535, 100.2856) ccw projected
  arc A3 (22.2896, 86.0447) -> (22.3201, 73.9669) centre (36.0355, 80.0405) ccw projected
  point P0 (0, 0)
extrude "Extrusion49" add sketch "Sketch53" along normal blind 10 and the other way blind 25
sketch "Sketch54" plane through (0, 0, 35) normal (0, 0, 1) x (1, 0, 0)
  line L0 (80, 35.3093) -> (80, 0) projected
  arc A0 (22.3201, 73.9669) -> (80, 35.3093) centre (81.7535, 100.2856) ccw projected
  arc A1 (22.2896, 86.0447) -> (22.3201, 73.9669) centre (36.0355, 80.0405) ccw projected
  arc A2 (80, 125) -> (22.2896, 86.0447) centre (81.8551, 60.0265) ccw projected
  line L1 (80, 160) -> (80, 125) projected
  arc A3 (80, 160) -> (80, 0) centre (80, 80) ccw projected
  point P0 (0, 0)
extrude "Extrusion50" cut sketch "Sketch54" against normal through all
sketch "Sketch55" plane through (0, 0, 15) normal (0, 0, -1) x (-1, 0, 0)
  arc A0 (-57.5, 120.2911) -> (-80, 125) centre (-81.8551, 60.0265) ccw projected
  line L0 (-80, 87.5) -> (-80, 125) projected
  line L1 (-73.8485, 87.5) -> (-80, 87.5) projected
  arc A1 (-57.5, 103.8485) -> (-73.8485, 87.5) centre (-50, 80) ccw projected
  line L2 (-57.5, 120.2911) -> (-57.5, 103.8485) projected
  arc A2 (-22.9467, 87.5) -> (-42.5, 111.7582) centre (-81.8551, 60.0265) ccw projected
  line L3 (-42.5, 103.8485) -> (-42.5, 111.7582) projected
  arc A3 (-26.1515, 87.5) -> (-42.5, 103.8485) centre (-50, 80) ccw projected
  line L4 (-22.9467, 87.5) -> (-26.1515, 87.5) projected
  arc A4 (-42.5, 48.4767) -> (-22.9916, 72.5) centre (-81.7535, 100.2856) ccw projected
  line L5 (-26.1515, 72.5) -> (-22.9916, 72.5) projected
  arc A5 (-42.5, 56.1515) -> (-26.1515, 72.5) centre (-50, 80) ccw projected
  line L6 (-42.5, 48.4767) -> (-42.5, 56.1515) projected
  arc A6 (-80, 35.3093) -> (-57.5, 39.98) centre (-81.7535, 100.2856) ccw projected
  line L7 (-57.5, 56.1515) -> (-57.5, 39.98) projected
  arc A7 (-73.8485, 72.5) -> (-57.5, 56.1515) centre (-50, 80) ccw projected
  line L8 (-80, 72.5) -> (-73.8485, 72.5) projected
  line L9 (-80, 35.3093) -> (-80, 72.5) projected
  point P0 (0, 0)
extrude "Extrusion51" add sketch "Sketch55" along normal blind 15
sketch "Sketch56" plane through (0, 0, 40) normal (0, 0, -1) x (-1, 0, 0)
  line L0 (-88, 72) -> (-110, 72)
  line L1 (-110, 72) -> (-110, 88)
  line L2 (-110, 88) -> (-88, 88)
  line L3 (-88, 88) -> (-88, 72)
  circle A0 centre (-100, 80) radius 6.5 projected
  circle A1 centre (-100, 80) radius 6.5 projected
  line L4 (-112, 65.5) -> (-88, 65.5) projected
  line L5 (-88, 65.5) -> (-88, 94.5) projected
  line L6 (-88, 94.5) -> (-112, 94.5) projected
  line L7 (-112, 94.5) -> (-112, 65.5) projected
  point P0 (0, 0)
  point P1 (-110, 80)
  dimension "d217" = 22
  dimension "d218" = 16
  dimension "d221" = 10
  constraints: 8 end point, 2 parallel, 1 horizontal, 1 horizontal alignment, 1 midpoint, 1 perpendicular
  measures "d217" distance of L1.end L2.end
  measures "d218" distance of L0.end L1.end
  measures "d221" distance from line of A0.centre L1
extrude "Extrusion52" add sketch "Sketch56" along normal blind 30 contours L5 L4 L7 L6 L2 L1 L0
sketch "Sketch57" plane through (0, 0, 50) normal (0, 0, 1) x (1, 0, 0)
  circle A0 centre (100, 80) radius 6.5 projected
  circle A1 centre (100, 80) radius 15
  point P0 (0, 0)
  dimension "d222" = 30
  constraints: 1 centre point, 1 coincident
  measures "d222" diameter of A1
extrude "Extrusion53" cut sketch "Sketch57" against normal blind 7
sketch "Sketch58" plane through (0, 0, 40) normal (0, 0, -1) x (-1, 0, 0)
  line L0 (-95, 10) -> (-95, 55.5) projected
  line L1 (-95, 55.5) -> (-150, 55.5) projected
  line L2 (-150, 10) -> (-150, 55.5) projected
  line L3 (-95, 10) -> (-150, 10) projected
  point P0 (0, 0)
extrude "Extrusion54" add sketch "Sketch58" along normal blind 32
sketch "Sketch59" plane through (130, 0, 8) normal (0, 0, -1) x (-1, 0, 0)
  line L0 (0, 0) -> (0, 10) projected
  line L1 (10, 0) -> (0, 0) projected
  line L2 (10, 0) -> (10, 10) projected
  line L3 (35, 10) -> (10, 10) projected
  line L4 (35, 55.5) -> (35, 10) projected
  line L5 (34, 55.5) -> (35, 55.5) projected
  line L6 (34, 55.5) -> (19, 55.5) projected
  line L7 (-20, 55.5) -> (19, 55.5) projected
  line L8 (-20, 10) -> (-20, 55.5) projected
  line L9 (0, 10) -> (-20, 10) projected
  point P0 (130, 0)
extrude "Extrusion55" add sketch "Sketch59" along normal blind 8
sketch "Sketch60" plane through (111, 104.5, 10) normal (0, 0, -1) x (-1, 0, 0)
  line L0 (15, -39) -> (15, -49) projected
  line L1 (0, -39) -> (0, -49) projected
  line L2 (15, -39) -> (0, -39)
  line L3 (0, -39) -> (0, -49)
  line L4 (0, -49) -> (15, -49)
  line L5 (15, -49) -> (15, -39)
  line L6 (-1, -10) -> (0, -10) projected
  line L7 (0, -39) -> (-1, -39)
  line L8 (-1, -39) -> (-1, -10)
  line L9 (-1, -10) -> (0, -10)
  line L10 (0, -10) -> (0, -39)
  line L11 (23, -39) -> (0, -39)
  line L12 (0, -39) -> (0, -32.5)
  line L13 (0, -32.5) -> (23, -32.5)
  line L14 (23, -32.5) -> (23, -39)
  point P0 (111, -104.5)
  point P1 (1, -32.5)
  constraints: 24 end point, 6 parallel, 3 horizontal, 3 perpendicular, 2 point on line, 1 coincident, 1 horizontal alignment
extrude "Extrusion56" add sketch "Sketch60" along normal blind 10
sketch "Sketch61" plane through (0, 0, 40) normal (0, 0, -1) x (-1, 0, 0)
  line L0 (-150, 104.5) -> (-95, 104.5) projected
  line L1 (-95, 104.5) -> (-95, 150) projected
  line L2 (-150, 150) -> (-95, 150) projected
  line L3 (-150, 104.5) -> (-150, 150) projected
  point P0 (0, 0)
extrude "Extrusion57" add sketch "Sketch61" along normal blind 30
body "Solid1"
